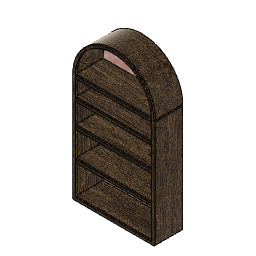
model (Autodesk Fusion 360 design; units mm, degrees)
Autodesk Fusion 360 part; units mm, degrees
sketch "front" plane through (0, 0, 0) normal (0, 1, 0) x (1, 0, 0) in component "bookshelf"
  line L0 (0, 0) -> (0, -1200)
  arc A0 (0, -1200) -> (900, -1200) centre (450, -1200) ccw
  line L1 (900, -1200) -> (900, 0)
  line L2 (900, 0) -> (0, 0)
  line L3 (450, -1200) -> (450, -1650) construction
  line L4 (18, -18) -> (18, -1200)
  arc A1 (18, -1200) -> (882, -1200) centre (450, -1200) ccw
  line L5 (882, -1200) -> (882, -18)
  line L6 (882, -18) -> (18, -18)
  line L7 (882, -18) -> (882, 0)
  line L8 (18, -18) -> (18, 0)
  line L9 (18, -1200) -> (882, -1199.9999)
  line L10 (882, -1199.9999) -> (882, -1181.9999)
  line L11 (882, -1181.9999) -> (18, -1181.9999)
  line L12 (18, -1181.9999) -> (18, -1200)
  line L13 (18, -981.9999) -> (882, -981.9999)
  line L14 (882, -981.9999) -> (882, -963.9999)
  line L15 (882, -963.9999) -> (18, -963.9999)
  line L16 (18, -963.9999) -> (18, -981.9999)
  line L17 (18, -713.9999) -> (882, -713.9999)
  line L18 (882, -713.9999) -> (882, -695.9999)
  line L19 (882, -695.9999) -> (18, -695.9999)
  line L20 (18, -695.9999) -> (18, -713.9999)
  line L21 (18, -30) -> (882, -30)
  line L22 (882, -30) -> (882, -12)
  line L23 (882, -12) -> (18, -12)
  line L24 (18, -12) -> (18, -30)
  line L25 (450, -1181.9999) -> (450, -981.9999) construction
  line L26 (450, -963.9999) -> (450, -713.9999) construction
  line L27 (450, -377.9999) -> (450, -30) construction
  line L28 (18, -395.9999) -> (882, -395.9999)
  line L29 (882, -395.9999) -> (882, -377.9999)
  line L30 (882, -377.9999) -> (18, -377.9999)
  line L31 (18, -377.9999) -> (18, -395.9999)
  line L32 (450, -395.9999) -> (450, -695.9999) construction
  dimension "d4" = 900
  dimension "d5" = 1650
  dimension "d8" = 18
  dimension "d27" = 30
  dimension "d28" = 200
  dimension "d29" = 250
  dimension "d30" = 300
  dimension "d31" = 347.9999
  dimension "d35" = 1181.9999
  constraint coincident L0.start L2.end
  constraint vertical L0
  constraint tangent L0 A0
  constraint parallel L0 L1
  constraint perpendicular L0 L2
  constraint tangent A0 L1
  constraint coincident A0.centre L3.start
  constraint midpoint A0 L3.end
  constraint coincident L2 L7.end
  constraint perpendicular L2 L7
  constraint coincident L2 L8.end
  constraint perpendicular L2 L8
  constraint horizontal L9
  constraint vertical L10
  constraint horizontal L11
  constraint vertical L12
  constraint coincident L5 L10.end
  constraint horizontal L13
  constraint vertical L14
  constraint horizontal L15
  constraint vertical L16
  constraint coincident L5 L14.end
  constraint coincident L4 L13.start
  constraint horizontal L17
  constraint vertical L18
  constraint horizontal L19
  constraint vertical L20
  constraint coincident L5 L18.end
  constraint coincident L4 L17.start
  constraint horizontal L21
  constraint vertical L22
  constraint horizontal L23
  constraint vertical L24
  constraint coincident L5 L22.end
  constraint coincident L4 L21.start
  constraint equal L10 L14
  constraint equal L14 L18
  constraint equal L18 L22
  constraint midpoint L11 L25.start
  constraint midpoint L13 L25.end
  constraint midpoint L15 L26.start
  constraint midpoint L17 L26.end
  constraint midpoint L21 L27.end
  constraint horizontal L28
  constraint vertical L29
  constraint horizontal L30
  constraint vertical L31
  constraint coincident L5 L29.end
  constraint coincident L4 L28.start
  constraint equal L18 L29
  constraint midpoint L27.start L30
  constraint midpoint L28 L32.start
  constraint midpoint L19 L32.end
  measures "d4" distance of L1.end L0.start
  measures "d5" distance of L2 L3.end
  measures "d8" distance of L21.end L22.end
  measures "d27" distance of L2 L21
  measures "d28" distance of L25.start L25.end
  measures "d29" distance of L26.start L26.end
  measures "d30" distance of L32.start L32.end
  measures "d31" distance of L27.start L27.end
  measures "d35" distance of L0.start L11
extrude "Extrude1" add sketch "front" against normal blind 300 contours L0 A0 L1 L2 L4 A1 L5 L7 L8 L10 L12 L14 L16 L18 L20 L22 L24 L29 L31 makes body 1 in component "bookshelf"
extrude "Extrude2" add sketch "front" against normal up to surface (300 mm away) separate body contours L6 L7 L8 L22 L23 L24 | L4 L5 L6 L21 L22 L24 | L4 L5 L28 L29 L30 L31 | L4 L5 L17 L18 L19 L20 | L4 L5 L13 L14 L15 L16 | L4 L5 L9 L10 L11 L12 makes body 2 at (594, -200, 963.9999) makes body 3 at (594, -200, 695.9999) makes body 4 at (594, -200, 1181.9999) makes body 5 at (594, -200, 12) makes body 6 at (594, -200, 377.9999) in component "bookshelf"
ref_plane "WorkPlane1" through (450, -150, 1181.9999) normal (0, 0, -1) x (1, 0, 0) in component "bookshelf"
split "Split1" by plane through (450, -150, 1181.9999) normal (0, 0, -1) bodies 1 makes body 7 at (0, -100, 394) makes body 8 at (900, -100, 788) in component "bookshelf"
extrude "Extrude4" add sketch "front" along normal blind 6 separate body contours L4 L5 L21 L30 | L4 L5 L28 L29 L30 L31 | L4 L5 L19 L28 | L4 L5 L17 L18 L19 L20 | L4 L5 L15 L17 | L4 L5 L13 L14 L15 L16 | L4 L5 L11 L13 | L4 L5 L9 L10 L11 L12 | A1 L9 makes body 9 in component "bookshelf"
sketch "edge" plane through (0, -300, 0) normal (0, -1, 0) x (1, 0, 0) in component "bookshelf"
  line L0 (18, 1181.9999) -> (0, 1181.9999)
  line L1 (0, 1181.9999) -> (0, 0)
  line L2 (0, 0) -> (18, 0)
  line L3 (18, 0) -> (18, 1181.9999)
  arc A0 (900, 1200) -> (0, 1200) centre (450, 1200) ccw
  line L4 (0, 0) -> (0, 1200)
  line L5 (900, 1200) -> (900, 0)
  line L6 (900, 0) -> (0, 0)
  line L7 (870, 30) -> (30, 30)
  line L8 (30, 30) -> (30, 1200)
  arc A1 (870, 1200) -> (30, 1200) centre (450, 1200) ccw
  line L9 (870, 1200) -> (870, 30)
  line L10 (18, 1200) -> (882, 1199.9999)
  line L11 (18, 981.9999) -> (882, 981.9999)
  line L12 (18, 713.9999) -> (882, 713.9999)
  line L13 (18, 395.9999) -> (882, 395.9999)
  line L14 (30, 1200) -> (870, 1200)
  line L15 (870, 1200) -> (870, 1170)
  line L16 (870, 1170) -> (30, 1170)
  line L17 (30, 1170) -> (30, 1200)
  line L18 (30, 981.9999) -> (870, 981.9999)
  line L19 (870, 981.9999) -> (870, 951.9999)
  line L20 (870, 951.9999) -> (30, 951.9999)
  line L21 (30, 951.9999) -> (30, 981.9999)
  line L22 (30, 713.9999) -> (870, 713.9999)
  line L23 (870, 713.9999) -> (870, 683.9999)
  line L24 (870, 683.9999) -> (30, 683.9999)
  line L25 (30, 683.9999) -> (30, 713.9999)
  line L26 (30, 395.9999) -> (870, 395.9999)
  line L27 (870, 395.9999) -> (870, 365.9999)
  line L28 (870, 365.9999) -> (30, 365.9999)
  line L29 (30, 365.9999) -> (30, 395.9999)
  dimension "d24" = 30
  dimension "d32" = 30
  constraint horizontal L14
  constraint vertical L15
  constraint horizontal L16
  constraint vertical L17
  constraint coincident L9 L15.end
  constraint horizontal L18
  constraint vertical L19
  constraint horizontal L20
  constraint vertical L21
  constraint coincident L9 L19.end
  constraint coincident L11 L18.start
  constraint coincident L8 L18.start
  constraint horizontal L22
  constraint vertical L23
  constraint horizontal L24
  constraint vertical L25
  constraint coincident L9 L23.end
  constraint coincident L12 L22.start
  constraint coincident L8 L22.start
  constraint horizontal L26
  constraint vertical L27
  constraint horizontal L28
  constraint vertical L29
  constraint coincident L9 L27.end
  constraint coincident L13 L26.start
  constraint coincident L8 L26.start
  constraint equal L15 L19
  constraint equal L19 L23
  constraint equal L23 L27
  measures "d32" distance of L26.end L27.end
extrude "Extrude5" add sketch "edge" along normal blind 18 separate body contours L0 L1 L2 L3 L4 L6 | L0 L3 A0 L4 L5 L6 L7 L8 A1 L9 L11 L13 L15 L17 L19 L23 L27 L29 | L3 L8 L11 L12 L21 | L3 L8 L12 L13 L25 makes body 10 in component "bookshelf"
extrude "Extrude6" add sketch "edge" along normal up to surface (18 mm away) separate body contours L8 L9 L11 L18 L19 L20 L21 | L8 L9 L12 L22 L23 L24 L25 | L8 L9 L10 L14 L15 L16 L17 | L8 L9 L13 L26 L27 L28 L29 makes body 11 at (310, -300, 971.9999) makes body 12 at (310, -300, 703.9999) makes body 13 at (310, -300, 1190) makes body 14 at (310, -300, 385.9999) in component "bookshelf"
component "bookshelf" placed x (1, 0, 0) y (0, 1, 0) z (0, 0, 1) at (0, 0, 0)
equation "height = 1650 mm"
equation "depth = 300 mm"
equation "width = 900 mm"
equation "d4 = width"
equation "d5 = height"
equation "plyT = 18 mm"
equation "d7 = -plyT"
equation "d8 = plyT"
equation "d12 = -depth"
equation "edge = 30 mm"
equation "d24 = edge"
equation "d25 = plyT"
equation "d27 = edge"
equation "d29 = d28 + 50 mm"
equation "d30 = d29 + 50 mm"
equation "d32 = edge"
